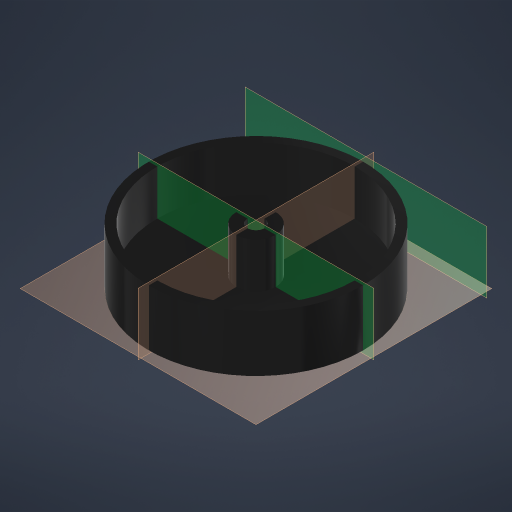
# Autodesk Inventor part: Wheel
Saved by Autodesk Inventor 2024 (Build 280153000, 153)
## iProperties
Manager: Louis Van Roosmaelen
Company: DCS - DIGITAL COMBAT SIMULATOR
Created: 2023-12-09
Part Number: Wheel
Material: S235
Catalog Web Link: http://emmausbovenbouw.op-weg.be/
Vendor: Emmaüsinstituut Bovenbouw Aalter
Document SubType Name: Modeling
Designer: Louis
Engineer: Declercq St.
Manufacturer: Standard
Standards Organization: Custom
Density: 7.86 g/cm^3
Appearance: Smooth - Black
IDENT.NR.: AJ2022
TEAM: 30
Title: F18C Home Cockpit
Author: Louis
Keywords: Ø
Autodesk Inventor part; units mm, degrees
sketch "Sketch1" plane through (0, 0, 0) normal (0, 0, 1) x (1, 0, 0)
  line L0 (0, 2.8582) -> (0, -2.8582) construction
  line L1 (-5.7775, 0) -> (5.7775, 0) construction
  circle A0 centre (0, 0) radius 1.5
  circle A1 centre (0, 0) radius 17.5
  circle A2 centre (0, 0) radius 3.5
  circle A3 centre (0, 0) radius 19
  dimension "d0" = 3
  dimension "d1" = 35
  dimension "d2" = 7
  dimension "d3" = 38
  constraints: 5 coincident, 4 centre point, 4 end point, 2 midpoint, 1 horizontal, 1 vertical
  measures "d0" diameter of A0
  measures "d1" diameter of A1
  measures "d2" diameter of A2
  measures "d3" diameter of A3
extrude "Extrusion1" add sketch "Sketch1" along normal blind 10
sketch "Sketch2" plane through (0, 0, 0) normal (0, 0, -1) x (-1, 0, 0)
  circle A0 centre (0, 0) radius 1.5 projected
  circle A1 centre (0, 0) radius 3.5 projected
  circle A2 centre (0, 0) radius 17.5 projected
  circle A3 centre (0, 0) radius 19 projected
extrude "Extrusion2" add sketch "Sketch2" against normal blind 2 contours A2
ref_plane "Ground" through (0, 19.5, 0) normal (0, 1, 0) x (-1, 0, 0)
body "Solid1"
